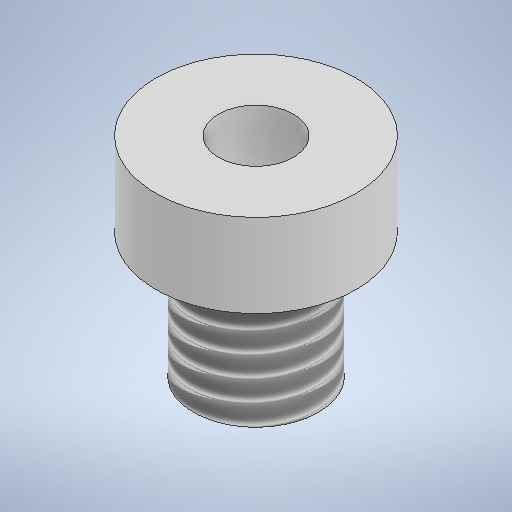
# Autodesk Inventor part: Part8
Saved by Autodesk Inventor 2025 (Build 290162000, 162)
## iProperties
Created: 2026-06-20
Part Number: Part8
Material: Generic
Document SubType Name: Modeling
Designer: saket
Density: 1 g/cm^3
Appearance: Default
Author: saket
Autodesk Inventor part; units mm, degrees
ref_plane "YZ Plane" through (0, 0, 0) normal (1, 0, 0) x (0, 1, 0)
ref_plane "XZ Plane" through (0, 0, 0) normal (0, 1, 0) x (-1, 0, 0)
ref_plane "XY Plane" through (0, 0, 0) normal (0, 0, 1) x (1, 0, 0)
sketch "Sketch1" plane through (0, 0, 0) normal (0, 1, 0) x (-1, 0, 0)
  circle A0 centre (0, 0) radius 2.25
  circle A1 centre (0, 0) radius 3.75
  circle A2 centre (0, 0) radius 6
  dimension "d0" = 4.5
  dimension "d1" = 7.5
  dimension "d2" = 12
  constraints: 3 centre point, 3 coincident
  measures "d0" diameter of A0
  measures "d1" diameter of A1
  measures "d2" diameter of A2
extrude "Extrusion1" add sketch "Sketch1" against normal blind 12.5 contours A1
extrude "Extrusion2" add sketch "Sketch1" against normal blind 5 contours A2
thread "Thread1" size "M8x1.25" class "6g" standard "ANSI Metric M Profile" length 10
body "Solid1"
